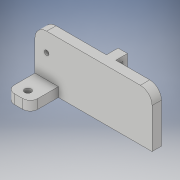
# Autodesk Inventor part: POE mounting for box
Saved by Autodesk Inventor 2018 (Build 220112000, 112)
## iProperties
Created: 2019-09-30
Part Number: POE mounting for box
Material: Generic
Document SubType Name: Modeling
Designer: Jacob
Density: 1 g/cm^3
Appearance: Default
Author: Jacob
Autodesk Inventor part; units mm, degrees
ref_plane "YZ Plane" through (0, 0, 0) normal (1, 0, 0) x (0, 1, 0)
ref_plane "XZ Plane" through (0, 0, 0) normal (0, 1, 0) x (-1, 0, 0)
ref_plane "XY Plane" through (0, 0, 0) normal (0, 0, 1) x (1, 0, 0)
sketch "Sketch1" plane through (0, 0, 0) normal (0, 1, 0) x (-1, 0, 0)
  line L0 (25, 2) -> (-25, 2)
  line L1 (-25, 2) -> (-25, -2)
  line L2 (-25, -2) -> (25, -2)
  line L3 (25, -2) -> (25, 2)
  line L4 (25, 2) -> (-25, -2) construction
  line L5 (-25, 2) -> (25, -2) construction
  point P0 (0, 0)
  dimension "d0" = 4
  dimension "d1" = 50
  constraints: 12 end point, 2 midpoint, 2 parallel, 1 horizontal, 1 perpendicular
  measures "d0" distance of L2.end L0.start
  measures "d1" distance of L1.end L2.end
extrude "Extrusion1" add sketch "Sketch1" along normal blind 20
fillet "Fillet1" radius 5 2 edges at (-25, 20, 0) (25, 20, 0)
sketch "Sketch2" plane through (-25, 0, 2) normal (0, 0, 1) x (1, 0, 0)
  line L0 (0, 0) -> (50, 0) projected
  arc A0 (5, 20) -> (0, 15) centre (5, 15) ccw projected
  line L1 (0, 15) -> (0, 0)
  line L2 (5, 20) -> (5, 0) construction
  circle A1 centre (5, 12) radius 1
  point P0 (25, 0)
  dimension "d44" = 12
  dimension "d45" = 2
  constraints: 4 end point, 3 point on line, 1 centre point, 1 perpendicular, 1 vertical
  measures "d44" distance from line of L0 A1.centre
  measures "d45" diameter of A1
extrude "Extrusion2" cut sketch "Sketch2" against normal blind 15
sketch "Sketch3" plane through (0, 0, 0) normal (0, -1, 0) x (1, 0, 0)
  line L0 (25, -2) -> (-25, -2) projected
  line L1 (25, 2) -> (-25, 2)
  line L2 (-25, 2) -> (-25, -2)
  line L3 (-25, -2) -> (25, -2)
  line L4 (25, -2) -> (25, 2)
  line L5 (25, 2) -> (-25, -2) construction
  line L6 (-25, 2) -> (25, -2) construction
  point P0 (0, 0)
  constraints: 12 end point, 2 midpoint, 2 parallel, 1 horizontal, 1 perpendicular
extrude "Extrusion3" add sketch "Sketch3" along normal blind 2
sketch "Sketch8" plane through (-20, 20, 2) normal (0, 0, 1) x (1, 0, 0)
  line L0 (-5, -5) -> (-5, -22) projected
  line L1 (-5, -22) -> (5, -22)
  line L2 (5, -22) -> (5, -18)
  line L3 (5, -18) -> (-5, -18)
  line L4 (-5, -18) -> (-5, -22)
  point P0 (20, -20)
  dimension "d36" = 4
  dimension "d37" = 10
  constraints: 8 end point, 2 parallel, 1 horizontal, 1 perpendicular
  measures "d36" distance of L1.end L2.end
  measures "d37" distance of L2.end L3.end
extrude "Extrusion9" add sketch "Sketch8" along normal blind 12
sketch "Sketch9" plane through (-25, 2, 2) normal (0, 1, 0) x (1, 0, 0)
  line L0 (10, -12) -> (0, -12) projected
  line L1 (5, -12) -> (5, 0) construction
  line L2 (0, 0) -> (10, 0) projected
  circle A0 centre (5, -8) radius 1.3907
  point P0 (25, 2)
  dimension "d40" = 4
  constraints: 2 end point, 2 midpoint, 1 centre point, 1 point on line
  measures "d40" distance from line of L0 A0.centre
extrude "Extrusion10" cut sketch "Sketch9" against normal blind 12
fillet "Fillet4" radius 3.175 2 edges at (-25, 0, 14) (-15, 0, 14)
sketch "Sketch10" plane through (20, 20, -2) normal (0, 0, -1) x (-1, 0, 0)
  line L0 (40, 0) -> (0, 0) projected
  line L1 (16.5, 0) -> (16.5, -22) construction
  line L2 (45, -22) -> (-5, -22) projected
  circle A0 centre (40, -8) radius 1 projected
  line L3 (14.5, 0) -> (18.5, 0)
  line L4 (18.5, 0) -> (18.5, -2)
  line L5 (18.5, -2) -> (14.5, -2)
  line L6 (14.5, -2) -> (14.5, 0)
  line L7 (14.5, 0) -> (18.5, -2) construction
  line L8 (18.5, 0) -> (14.5, -2) construction
  point P0 (20, -20)
  point P1 (16.5, -1)
  dimension "d46" = 23.5
  dimension "d47" = 0
  dimension "d48" = 2
  dimension "d51" = 4
  constraints: 14 end point, 3 point on line, 2 midpoint, 2 parallel, 1 horizontal, 1 perpendicular, 1 vertical
  measures "d46" distance from line of L1 A0.centre
  measures "d47" distance between parallel lines of L0 L3
  measures "d48" distance of L3.end L4.end
  measures "d51" distance of L4.end L5.end
extrude "Extrusion11" add sketch "Sketch10" along normal blind 5 contours L4 L5 L6 L0
sketch "Sketch11" plane through (1.5, 18, -2) normal (0, -1, 0) x (1, 0, 0)
  line L0 (4, -5) -> (0, -5) projected
  line L1 (0, 0) -> (0, -5) projected
  line L2 (4, -5) -> (0, -5)
  line L3 (0, -5) -> (0, -3)
  line L4 (0, -3) -> (4, -3)
  line L5 (4, -3) -> (4, -5)
  point P0 (-1.5, 2)
  dimension "d52" = 2
  constraints: 8 end point, 2 parallel, 1 horizontal, 1 perpendicular, 1 point on line
  measures "d52" distance between parallel lines of L0 L4
extrude "Extrusion12" add sketch "Sketch11" along normal blind 20
sketch "Sketch12" plane through (25, -2, -2) normal (0, 0, -1) x (-1, 0, 0)
  line L0 (23.5, 20) -> (19.5, 20) projected
  line L1 (21.5, 20) -> (21.5, 0) construction
  line L2 (50, 0) -> (0, 0) projected
  circle A0 centre (21.5, 2) radius 1
  point P0 (25, 2)
  dimension "d57" = 2
  dimension "d58" = 2
  constraints: 2 end point, 2 point on line, 1 centre point, 1 midpoint, 1 vertical
  measures "d57" diameter of A0
  measures "d58" distance from line of L2 A0.centre
extrude "Extrusion13" cut sketch "Sketch12" against normal blind 3
sketch "Sketch13" plane through (25, -2, -2) normal (0, 0, -1) x (-1, 0, 0)
  circle A0 centre (21.5, 2) radius 1 projected
  circle A1 centre (21.5, 2) radius 2
  point P0 (25, 2)
  dimension "d61" = 4
  constraints: 1 centre point, 1 coincident
  measures "d61" diameter of A1
extrude "Extrusion14" add sketch "Sketch13" along normal blind 2.5
sketch "Sketch14" plane through (20, 20, -7) normal (0, 0, -1) x (-1, 0, 0)
  line L0 (45, -22) -> (16.5, -22) projected
  line L1 (16.5, -22) -> (16.5, -16.8433) construction
  circle A0 centre (16.5, -20) radius 1 projected
  circle A1 centre (16.5, -20) radius 1
  point P0 (20, -20)
  dimension "d64" = 2
  constraints: 2 end point, 1 centre point, 1 coincident, 1 vertical
  measures "d64" diameter of A1
extrude "Extrusion15" cut sketch "Sketch14" against normal blind 2.5
body "Solid1"
